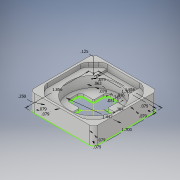
# Autodesk Inventor part: SnakeControllerCase_v3
Saved by Autodesk Inventor 2019.1 (Build 231200000, 200)
## iProperties
Created: 2018-11-28
Part Number: SnakeControllerCase_v3
Material: Generic
Document SubType Name: Modeling
Designer: Edward Hughes
Density: 1 g/cm^3
Appearance: Default
Author: Edward Hughes
Autodesk Inventor part; units mm, degrees
ref_plane "YZ Plane" through (0, 0, 0) normal (1, 0, 0) x (0, 1, 0)
ref_plane "XZ Plane" through (0, 0, 0) normal (0, 1, 0) x (-1, 0, 0)
ref_plane "XY Plane" through (0, 0, 0) normal (0, 0, 1) x (1, 0, 0)
sketch "Sketch1" plane through (0, 0, 0) normal (0, 1, 0) x (-1, 0, 0)
  circle A0 centre (0, 0) radius 18.3769
  line L0 (18.3769, 18.3769) -> (-18.3769, -18.3769) construction
  line L1 (-18.3769, 18.3769) -> (18.3769, -18.3769) construction
  line L2 (13.335, 21.59) -> (-13.335, 21.59)
  line L3 (-21.59, 13.335) -> (-21.59, -13.335)
  line L4 (-13.335, -21.59) -> (13.335, -21.59)
  line L5 (21.59, -13.335) -> (21.59, 13.335)
  line L6 (21.59, 21.59) -> (-21.59, -21.59) construction
  line L7 (-21.59, 21.59) -> (21.59, -21.59) construction
  line L8 (21.59, 13.335) -> (13.335, 21.59)
  line L9 (-13.335, 21.59) -> (-21.59, 13.335)
  line L10 (-21.59, -13.335) -> (-13.335, -21.59)
  line L11 (13.335, -21.59) -> (21.59, -13.335)
  circle A1 centre (15.24, -15.24) radius 1.0033
  circle A2 centre (-15.24, -15.24) radius 1.0033
  circle A3 centre (-15.24, 15.24) radius 1.0033
  circle A4 centre (15.24, 15.24) radius 1.0033
  line L12 (11.9917, -21.9869) -> (-11.9917, -21.9869)
  line L13 (-21.9869, -11.9917) -> (-21.9869, 11.9917)
  line L14 (-11.9917, 21.9869) -> (11.9917, 21.9869)
  line L15 (21.9869, 11.9917) -> (21.9869, -11.9917)
  line L16 (-20.3962, 23.5712) -> (20.3962, 23.5712)
  line L17 (23.5712, 20.3962) -> (23.5712, -20.3962)
  line L18 (20.3962, -23.5712) -> (-20.3962, -23.5712)
  line L19 (-23.5712, -20.3962) -> (-23.5712, 20.3962)
  line L20 (-23.5712, 23.5712) -> (23.5712, -23.5712) construction
  line L21 (23.5712, 23.5712) -> (-23.5712, -23.5712) construction
  arc A5 (20.3962, -23.5712) -> (23.5712, -20.3962) centre (20.3962, -20.3962) ccw
  arc A6 (-23.5712, -20.3962) -> (-20.3962, -23.5712) centre (-20.3962, -20.3962) ccw
  arc A7 (-20.3962, 23.5712) -> (-23.5712, 20.3962) centre (-20.3962, 20.3962) ccw
  arc A8 (23.5712, 20.3962) -> (20.3962, 23.5712) centre (20.3962, 20.3962) ccw
  circle A9 centre (20.3962, -20.3962) radius 1.0033
  circle A10 centre (-20.3962, -20.3962) radius 1.0033
  circle A11 centre (-20.3962, 20.3962) radius 1.0033
  circle A12 centre (20.3962, 20.3962) radius 1.0033
  line L22 (16.4818, -20.127) -> (20.127, -16.4818)
  line L23 (20.127, 16.4818) -> (16.4818, 20.127)
  line L24 (-16.4818, 20.127) -> (-20.127, 16.4818)
  line L25 (-20.127, -16.4818) -> (-16.4818, -20.127)
  arc A13 (21.9869, 11.9917) -> (20.127, 16.4818) centre (15.6369, 11.9917) ccw
  arc A14 (16.4818, 20.127) -> (11.9917, 21.9869) centre (11.9917, 15.6369) ccw
  arc A15 (-11.9917, 21.9869) -> (-16.4818, 20.127) centre (-11.9917, 15.6369) ccw
  arc A16 (-20.127, 16.4818) -> (-21.9869, 11.9917) centre (-15.6369, 11.9917) ccw
  arc A17 (-21.9869, -11.9917) -> (-20.127, -16.4818) centre (-15.6369, -11.9917) ccw
  arc A18 (-16.4818, -20.127) -> (-11.9917, -21.9869) centre (-11.9917, -15.6369) ccw
  arc A19 (11.9917, -21.9869) -> (16.4818, -20.127) centre (11.9917, -15.6369) ccw
  arc A20 (20.127, -16.4818) -> (21.9869, -11.9917) centre (15.6369, -11.9917) ccw
  line L26 (4.3815, -5.969) -> (4.3815, -12.5476)
  line L27 (2.794, -14.1351) -> (-2.794, -14.1351)
  line L28 (-4.3815, -12.5476) -> (-4.3815, -5.969)
  line L29 (4.3815, 5.969) -> (4.3815, 12.5476)
  line L30 (2.794, 14.1351) -> (-2.794, 14.1351)
  line L31 (-4.3815, 12.5476) -> (-4.3815, 5.969)
  line L32 (-5.969, -4.3815) -> (-12.5476, -4.3815)
  line L33 (-14.1351, -2.794) -> (-14.1351, 2.794)
  line L34 (-12.5476, 4.3815) -> (-5.969, 4.3815)
  line L35 (5.969, -4.3815) -> (12.5476, -4.3815)
  line L36 (14.1351, -2.794) -> (14.1351, 2.794)
  line L37 (12.5476, 4.3815) -> (5.969, 4.3815)
  arc A21 (2.794, -14.1351) -> (4.3815, -12.5476) centre (2.794, -12.5476) ccw
  arc A22 (-4.3815, -12.5476) -> (-2.794, -14.1351) centre (-2.794, -12.5476) ccw
  arc A23 (-4.3815, -5.969) -> (-5.969, -4.3815) centre (-5.969, -5.969) ccw
  arc A24 (-14.1351, -2.794) -> (-12.5476, -4.3815) centre (-12.5476, -2.794) ccw
  arc A25 (-14.1351, -2.794) -> (-12.5476, -4.3815) centre (-12.5476, -2.794) ccw
  arc A26 (-12.5476, 4.3815) -> (-14.1351, 2.794) centre (-12.5476, 2.794) ccw
  arc A27 (-5.969, 4.3815) -> (-4.3815, 5.969) centre (-5.969, 5.969) ccw
  arc A28 (-2.794, 14.1351) -> (-4.3815, 12.5476) centre (-2.794, 12.5476) ccw
  arc A29 (4.3815, 12.5476) -> (2.794, 14.1351) centre (2.794, 12.5476) ccw
  arc A30 (4.3815, 5.969) -> (5.969, 4.3815) centre (5.969, 5.969) ccw
  arc A31 (14.1351, 2.794) -> (12.5476, 4.3815) centre (12.5476, 2.794) ccw
  arc A32 (12.5476, -4.3815) -> (14.1351, -2.794) centre (12.5476, -2.794) ccw
  arc A33 (5.969, -4.3815) -> (4.3815, -5.969) centre (5.969, -5.969) ccw
  line L38 (-2.794, -14.9289) -> (2.794, -14.9289)
  arc A34 (2.794, -14.9289) -> (5.1753, -12.5476) centre (2.794, -12.5476) ccw
  line L39 (5.1753, -12.5476) -> (5.1753, -5.969)
  arc A35 (5.969, -5.1753) -> (5.1753, -5.969) centre (5.969, -5.969) ccw
  line L40 (5.969, -5.1753) -> (12.5476, -5.1753)
  arc A36 (12.5476, -5.1753) -> (14.9289, -2.794) centre (12.5476, -2.794) ccw
  line L41 (14.9289, -2.794) -> (14.9289, 2.794)
  arc A37 (14.9289, 2.794) -> (12.5476, 5.1753) centre (12.5476, 2.794) ccw
  line L42 (12.5476, 5.1753) -> (5.969, 5.1753)
  arc A38 (5.1753, 5.969) -> (5.969, 5.1753) centre (5.969, 5.969) ccw
  line L43 (5.1753, 5.969) -> (5.1753, 12.5476)
  arc A39 (5.1753, 12.5476) -> (2.794, 14.9289) centre (2.794, 12.5476) ccw
  line L44 (2.794, 14.9289) -> (-2.794, 14.9289)
  arc A40 (-2.794, 14.9289) -> (-5.1753, 12.5476) centre (-2.794, 12.5476) ccw
  line L45 (-5.1753, 12.5476) -> (-5.1753, 5.969)
  arc A41 (-5.969, 5.1753) -> (-5.1753, 5.969) centre (-5.969, 5.969) ccw
  line L46 (-5.969, 5.1753) -> (-12.5476, 5.1753)
  arc A42 (-12.5476, 5.1753) -> (-14.9289, 2.794) centre (-12.5476, 2.794) ccw
  line L47 (-14.9289, 2.794) -> (-14.9289, -2.794)
  arc A43 (-14.9289, -2.794) -> (-12.5476, -5.1753) centre (-12.5476, -2.794) ccw
  line L48 (-12.5476, -5.1753) -> (-5.969, -5.1753)
  arc A44 (-5.1753, -5.969) -> (-5.969, -5.1753) centre (-5.969, -5.969) ccw
  line L49 (-5.1753, -5.969) -> (-5.1753, -12.5476)
  arc A45 (-5.1753, -12.5476) -> (-2.794, -14.9289) centre (-2.794, -12.5476) ccw
  line L50 (11.9917, -21.59) -> (-11.9917, -21.59)
  line L51 (-11.9917, -21.59) -> (-11.9917, -13.9252)
  line L52 (11.9917, -13.9252) -> (11.9917, -21.59)
  point P0 (4.3815, -14.1351)
  point P1 (-4.3815, -14.1351)
  point P2 (4.3815, 14.1351)
  point P3 (-14.1351, 4.3815)
  point P4 (-4.3815, 4.3815)
  point P5 (14.1351, 4.3815)
  point P6 (4.3815, 4.3815)
  dimension "d33" = 36.7538
  dimension "d34" = 43.18
  dimension "d35" = 43.18
  dimension "d48" = 2.0066
  dimension "d49" = 2.0066
  dimension "d50" = 2.0066
  dimension "d51" = 2.0066
  dimension "d52" = 0.3969
  dimension "d53" = 47.1424
  dimension "d54" = 47.1424
  dimension "d55" = 3.175
  dimension "d56" = 2.0066
  dimension "d57" = 2.0066
  dimension "d58" = 2.0066
  dimension "d59" = 2.0066
  dimension "d62" = 6.35
  dimension "d79" = 8.763
  dimension "d84" = 1.5875
  dimension "d85" = 0.7937
  dimension "d86" = 9.7536
  constraints: 106 end point, 74 point on circle, 50 tangent, 45 centre point, 25 point on line, 22 equal radius, 15 parallel, 8 perpendicular, 6 midpoint, 5 horizontal, 4 coincident, 26 other
  measures "d34" distance of L7.end L6.end
  measures "d35" distance of L6.end L7.start
  measures "d48" diameter of A1
  measures "d49" diameter of A2
  measures "d50" diameter of A3
  measures "d51" diameter of A4
  measures "d52" distance between parallel lines of L4 L12
  measures "d53" distance of L20.end L21.end
  measures "d54" distance of L21.start L20.end
  measures "d55" radius of A5
  measures "d56" diameter of A9
  measures "d57" diameter of A10
  measures "d58" diameter of A11
  measures "d59" diameter of A12
  measures "d62" radius of A13
  measures "d79" distance of point (4.381, -14.135) point (-4.381, -14.135)
  measures "d84" radius of A21
  measures "d85" distance between parallel lines of L27 L38
  measures "d86" distance between parallel lines of L27 L32
extrude "outer" add sketch "Sketch1" along normal blind 12.7 contours L16 A8 L17 A5 L18 A6 L19 A7
extrude "pcb support" add sketch "Sketch1" along normal blind 9.525 contours A0 L51 L4 L10 L3 L9 L2 L8 L5 L11 L52 | A0 L52 L4 L51 | L12 A18 L25 A17 L13 A16 L24 A15 L14 A14 L23 A13 L15 A20 L22 A19
extrude "pcb screw hole location" add sketch "Sketch1" along normal blind 9.525 contours A1 | A2 | A3 | A4
extrude "back cover screw hole location" add sketch "Sketch1" along normal blind 12.7 contours A9 | A10 | A11 | A12
extrude "dpad face" add sketch "Sketch1" along normal blind 1.5875 contours A0
sketch "Sketch3" plane through (20.3962, 0, -23.5712) normal (0, 0, -1) x (-1, 0, 0)
  line L0 (0, 0) -> (40.7924, 0) projected
  line L1 (-3.175, 0) -> (-3.175, 12.7) projected
  line L2 (32.3879, 9.525) -> (8.4045, 9.525) projected
  line L3 (8.4045, 9.525) -> (32.3879, 9.525) projected
  circle A0 centre (20.3962, 9.525) radius 3.9687
  point P0 (20.3962, 0)
  dimension "d92" = 7.9375
  constraints: 1 centre point, 1 coincident, 1 midpoint
  measures "d92" diameter of A0
extrude "ether cable" [suppressed]
sketch "Sketch4" plane through (0, 9.525, 0) normal (0, 1, 0) x (1, 0, 0)
  circle A0 centre (0, 0) radius 18.3769 projected
  line L0 (11.9917, 21.9869) -> (-11.9917, 21.9869) projected
  line L1 (-11.9917, 21.9869) -> (11.9917, 21.9869)
  line L2 (11.9917, 21.9869) -> (11.9917, 13.9252)
  line L3 (-11.9917, 13.9252) -> (-11.9917, 21.9869)
  arc A1 (11.9917, 13.9252) -> (-11.9917, 13.9252) centre (0, 0) ccw
  constraints: 6 end point, 2 point on circle, 1 centre point, 1 horizontal, 1 parallel, 1 perpendicular, 3 other
extrude "pocket" cut sketch "Sketch4" against normal blind 1.5875 contours A0 L3 L0 L2
body "Solid1"
